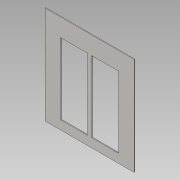
# Autodesk Inventor part: Interior Frame
Saved by Autodesk Inventor 2016 (Build 200138000, 138)
## iProperties
Created: 2017-05-19
Part Number: Interior Frame
Material: Generic
Document SubType Name: Modeling
Designer: 31745
Density: 1 g/cm^3
Appearance: Default
Author: 31745
Autodesk Inventor part; units mm, degrees
ref_plane "YZ Plane" through (0, 0, 0) normal (1, 0, 0) x (0, 1, 0)
ref_plane "XZ Plane" through (0, 0, 0) normal (0, 1, 0) x (-1, 0, 0)
ref_plane "XY Plane" through (0, 0, 0) normal (0, 0, 1) x (1, 0, 0)
sketch "Sketch1" plane through (0, 0, 0) normal (0, 0, 1) x (1, 0, 0)
  line L0 (0, 0) -> (254, 0)
  line L1 (254, 0) -> (254, 279.4)
  line L2 (254, 279.4) -> (0, 279.4)
  line L3 (0, 279.4) -> (0, 0)
  line L4 (44.45, 228.6) -> (120.65, 228.6)
  line L5 (120.65, 228.6) -> (120.65, 25.4)
  line L6 (120.65, 25.4) -> (44.45, 25.4)
  line L7 (44.45, 25.4) -> (44.45, 228.6)
  line L8 (133.35, 228.6) -> (209.55, 228.6)
  line L9 (209.55, 228.6) -> (209.55, 25.4)
  line L10 (209.55, 25.4) -> (133.35, 25.4)
  line L11 (133.35, 25.4) -> (133.35, 228.6)
  line L12 (120.65, 228.6) -> (133.35, 228.6)
  point P0 (127, 228.6)
  point P1 (127, 279.4)
  dimension "d0" = 254
  dimension "d1" = 279.4
  dimension "d2" = 12.7
  dimension "d3" = 76.2
  dimension "d4" = 76.2
  dimension "d5" = 50.8
  dimension "d6" = 25.4
  constraints: 26 end point, 6 parallel, 4 horizontal, 3 perpendicular, 2 midpoint, 2 point on line, 1 vertical alignment
  measures "d0" distance of L2.end L1.end
  measures "d1" distance of L1.end L0.end
  measures "d2" distance of L4.end L8.start
  measures "d3" distance of L8.start L8.end
  measures "d4" distance of L4.start L4.end
  measures "d5" distance between parallel lines of L2 L8
  measures "d6" distance between parallel lines of L0 L10
extrude "Extrusion1" add sketch "Sketch1" along normal blind 2.286
equation "\"d4\" = d3"
body "Solid1"
